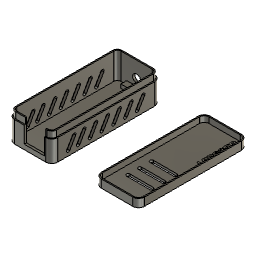
TubesZB_2022_PoE_Coordinator_Case_Rev_K_Olimex (Autodesk Fusion 360 design; units mm, degrees)
Autodesk Fusion 360 part; units mm, degrees
note: some values were not read from the file. Set by a fixed rule: which face or edge a step refers to.
sketch "Sketch1" plane through (0, 0, 0) normal (0, 0, 1) x (1, 0, 0)
  line L0 (0, 0) -> (36.6, 0)
  line L1 (36.6, 0) -> (36.6, 92.2)
  line L2 (36.6, 92.2) -> (0, 92.2)
  line L3 (0, 92.2) -> (0, 0)
  line L4 (105.8273, 96.6) -> (69.2273, 96.6)
  line L5 (69.2273, 4.4) -> (105.8273, 4.4)
  line L6 (105.8273, 4.4) -> (105.8273, 96.6)
  line L7 (69.2273, 96.6) -> (69.2273, 4.4)
  dimension "d1" = 36.6
  dimension "d2" = 92.2
  dimension "d3" = 36.6
  dimension "d4" = 92.2
  constraint horizontal L0
  constraint vertical L1
  constraint horizontal L2
  constraint vertical L3
  constraint coincident L0.start L3.end
  constraint horizontal L5
  constraint vertical L6
  constraint horizontal L4
  constraint vertical L7
  measures "d1" distance of L0.start L0.end
  measures "d2" distance of L0.start L2.end
  measures "d3" distance of L5.start L5.end
  measures "d4" distance of L4.end L5.start
extrude "Extrude1" add sketch "Sketch1" along normal blind 18 contours L0 L1 L2 L3 makes body 1
sketch "Sketch2" plane through (0, 0, 0) normal (0, 0, 1) x (1, 0, 0)
extrude "Extrude2" add sketch "Sketch1" along normal blind 6.8 separate body contours L4 L5 L6 L7 makes body 2
fillet "Fillet1" radius 5 4 edges at (0, 0, 9) (36.6, 0, 9) (36.6, 92.2, 9) (0, 92.2, 9) on bodies 1
fillet "Fillet2" radius 5 4 edges at (105.8273, 4.4, 3.4) (69.2273, 4.4, 3.4) (105.8273, 96.6, 3.4) (69.2273, 96.6, 3.4) on bodies 2
shell "Shell1" thickness 1 removed faces 1 at (93.6273, 36.8, 6.8) on bodies 2
shell "Shell2" thickness 1 removed faces 1 at (12.2, 59.8, 18) on bodies 1
extrude "Extrude3" cut 1 faces at (81.7606, 36.8, 1) along direction (0, 0, -1) blind 0.1 on bodies 2 bodies 2
extrude "Extrude4" add 1 faces at (12.5333, 59.8, 1) along direction (0, 0, 1) blind 22.2 on bodies 1 bodies 1
shell "Shell3" thickness 1 removed faces 1 at (12.5333, 59.8, 23.2) on bodies 1
extrude "Extrude5" cut 1 faces at (12.5333, 59.8, 1) along direction (0, 0, -1) blind 0.1 on bodies 1 bodies 1
sketch "Sketch3" plane through (36.6, 0, 0) normal (1, 0, 0) x (0, 1, 0)
  line L0 (87.2, 0) -> (87.2, 18)
  line L1 (87.2, 18) -> (5, 18)
  line L2 (5, 18) -> (5, 0)
  line L3 (5, 0) -> (87.2, 0)
  line L4 (15.2859, 3.55) -> (20.2859, 12.2103)
  arc A0 (20.2859, 12.2103) -> (17.6878, 13.7103) centre (18.9869, 12.9603) ccw
  line L5 (17.6878, 13.7103) -> (12.6878, 5.05)
  arc A1 (12.6878, 5.05) -> (15.2859, 3.55) centre (13.9869, 4.3) ccw
  line L6 (13.9869, 4.3) -> (18.9869, 12.9603) construction
  arc A2 (21.1822, 5.05) -> (23.7803, 3.55) centre (22.4812, 4.3) ccw
  arc A3 (28.7803, 12.2103) -> (26.1822, 13.7103) centre (27.4812, 12.9603) ccw
  line L7 (22.4812, 4.3) -> (27.4812, 12.9603) construction
  line L8 (23.7803, 3.55) -> (28.7803, 12.2103)
  line L9 (26.1822, 13.7103) -> (21.1822, 5.05)
  arc A4 (38.7803, 12.2103) -> (36.1822, 13.7103) centre (37.4812, 12.9603) ccw
  line L10 (33.7803, 3.55) -> (38.7803, 12.2103)
  line L11 (32.4812, 4.3) -> (37.4812, 12.9603) construction
  arc A5 (31.1822, 5.05) -> (33.7803, 3.55) centre (32.4812, 4.3) ccw
  line L12 (36.1822, 13.7103) -> (31.1822, 5.05)
  line L13 (43.7803, 3.55) -> (48.7803, 12.2103)
  line L14 (46.1822, 13.7103) -> (41.1822, 5.05)
  line L15 (42.4812, 4.3) -> (47.4812, 12.9603) construction
  arc A6 (41.1822, 5.05) -> (43.7803, 3.55) centre (42.4812, 4.3) ccw
  arc A7 (48.7803, 12.2103) -> (46.1822, 13.7103) centre (47.4812, 12.9603) ccw
  line L16 (53.7803, 3.55) -> (58.7803, 12.2103)
  arc A8 (51.1822, 5.05) -> (53.7803, 3.55) centre (52.4812, 4.3) ccw
  line L17 (52.4812, 4.3) -> (57.4812, 12.9603) construction
  arc A9 (58.7803, 12.2103) -> (56.1822, 13.7103) centre (57.4812, 12.9603) ccw
  line L18 (56.1822, 13.7103) -> (51.1822, 5.05)
  line L19 (63.7803, 3.55) -> (68.7803, 12.2103)
  line L20 (62.4812, 4.3) -> (67.4812, 12.9603) construction
  line L21 (66.1822, 13.7103) -> (61.1822, 5.05)
  arc A10 (68.7803, 12.2103) -> (66.1822, 13.7103) centre (67.4812, 12.9603) ccw
  arc A11 (61.1822, 5.05) -> (63.7803, 3.55) centre (62.4812, 4.3) ccw
  arc A12 (71.1822, 5.05) -> (73.7803, 3.55) centre (72.4812, 4.3) ccw
  arc A13 (78.7803, 12.2103) -> (76.1822, 13.7103) centre (77.4812, 12.9603) ccw
  line L22 (76.1822, 13.7103) -> (71.1822, 5.05)
  line L23 (73.7803, 3.55) -> (78.7803, 12.2103)
  line L24 (72.4812, 4.3) -> (77.4812, 12.9603) construction
  point P0 (38.7803, 12.2103)
  dimension "d22" = 10
  dimension "d23" = 3
  dimension "d24" = 10
  dimension "d25" = 3
  dimension "d26" = 10
  dimension "d27" = 3
  dimension "d28" = 10
  dimension "d29" = 3
  dimension "d30" = 10
  dimension "d31" = 3
  dimension "d32" = 10
  dimension "d33" = 3
  dimension "d34" = 10
  dimension "d35" = 3
  constraint tangent L4 A0
  constraint tangent A0 L5
  constraint parallel L4 L5
  constraint tangent L5 A1
  constraint tangent L4 A1
  constraint tangent A3 L8
  constraint tangent A3 L9
  constraint parallel L8 L9
  constraint tangent A2 L9
  constraint tangent A2 L8
  constraint tangent A4 L10
  constraint tangent A4 L12
  constraint parallel L10 L12
  constraint tangent A5 L12
  constraint tangent L10 A5
  constraint tangent L13 A7
  constraint tangent L14 A7
  constraint parallel L13 L14
  constraint tangent L14 A6
  constraint tangent L13 A6
  constraint tangent L16 A9
  constraint tangent A9 L18
  constraint parallel L16 L18
  constraint tangent A8 L18
  constraint tangent L16 A8
  constraint tangent L19 A10
  constraint tangent L21 A10
  constraint parallel L19 L21
  constraint tangent L21 A11
  constraint tangent L19 A11
  constraint tangent A13 L23
  constraint tangent A13 L22
  constraint parallel L22 L23
  constraint tangent A12 L22
  constraint tangent A12 L23
  measures "d22" distance of A1.centre A0.centre
  measures "d23" diameter of A0
  measures "d24" distance of A2.centre A3.centre
  measures "d25" diameter of A3
  measures "d26" distance of A4.centre L11.start
  measures "d27" diameter of A4
  measures "d28" distance of L15.start L15.end
  measures "d29" diameter of A7
  measures "d30" distance of L17.end A8.centre
  measures "d31" diameter of A9
  measures "d32" distance of L20.start L20.end
  measures "d33" diameter of A10
  measures "d34" distance of A12.centre A13.centre
  measures "d35" diameter of A13
extrude "Extrude13" cut sketch "Sketch3" against normal blind 59.488 contours L4 A0 L5 A1 | A2 A3 L8 L9 | A4 L10 A5 L12 | L13 L14 A6 A7 | L16 A8 A9 L18 | L19 L21 A10 A11 | A12 A13 L22 L23 bodies 1
sketch "Sketch4" plane through (0, 0, 0.9) normal (0, 0, 1) x (-1, 0, 0)
  arc A0 (-74.2273, -95.6) -> (-70.2273, -91.6) centre (-74.2273, -91.6) ccw
  line L0 (-70.2273, -91.6) -> (-70.2273, -9.4)
  arc A1 (-70.2273, -9.4) -> (-74.2273, -5.4) centre (-74.2273, -9.4) ccw
  line L1 (-74.2273, -5.4) -> (-100.8273, -5.4)
  arc A2 (-100.8273, -5.4) -> (-104.8273, -9.4) centre (-100.8273, -9.4) ccw
  line L2 (-104.8273, -9.4) -> (-104.8273, -91.6)
  arc A3 (-104.8273, -91.6) -> (-100.8273, -95.6) centre (-100.8273, -91.6) ccw
  line L3 (-100.8273, -95.6) -> (-74.2273, -95.6)
  line L4 (-77.8, -22.0707) -> (-97.8, -22.0707)
  arc A4 (-97.8, -22.0707) -> (-97.8, -25.0707) centre (-97.8, -23.5707) ccw
  line L5 (-97.8, -25.0707) -> (-77.8, -25.0707)
  arc A5 (-77.8, -25.0707) -> (-77.8, -22.0707) centre (-77.8, -23.5707) ccw
  line L6 (-77.8, -23.5707) -> (-97.8, -23.5707) construction
  line L7 (-77.8, -32.0707) -> (-97.8, -32.0707)
  arc A6 (-97.8, -32.0707) -> (-97.8, -35.0707) centre (-97.8, -33.5707) ccw
  line L8 (-97.8, -35.0707) -> (-77.8, -35.0707)
  arc A7 (-77.8, -35.0707) -> (-77.8, -32.0707) centre (-77.8, -33.5707) ccw
  line L9 (-77.8, -33.5707) -> (-97.8, -33.5707) construction
  line L10 (-77.8, -43.5707) -> (-97.8, -43.5707) construction
  line L11 (-97.8, -45.0707) -> (-77.8, -45.0707)
  arc A8 (-77.8, -45.0707) -> (-77.8, -42.0707) centre (-77.8, -43.5707) ccw
  line L12 (-77.8, -42.0707) -> (-97.8, -42.0707)
  arc A9 (-97.8, -42.0707) -> (-97.8, -45.0707) centre (-97.8, -43.5707) ccw
  constraint tangent L4 A4
  constraint tangent A4 L5
  constraint parallel L4 L5
  constraint tangent L5 A5
  constraint tangent L4 A5
  constraint horizontal L6
  constraint tangent L7 A6
  constraint tangent A6 L8
  constraint parallel L7 L8
  constraint tangent L8 A7
  constraint tangent L7 A7
  constraint horizontal L9
  constraint tangent L12 A9
  constraint tangent L11 A9
  constraint parallel L11 L12
  constraint tangent L11 A8
  constraint tangent A8 L12
  constraint horizontal L10
extrude "Extrude7" cut sketch "Sketch4" against normal blind 5 contours L4 A4 L5 A5 | L7 A6 L8 A7 | L11 A8 L12 A9 bodies 2
sketch "Sketch5" plane through (0, 0, 0) normal (0, 0, 1) x (1, 0, 0)
  line L0 (98.3981, 60.428) -> (98.2294, 82.6189) construction
  line L1 (98.2294, 82.6189) -> (102.261, 82.6495) construction
  line L2 (102.261, 82.6495) -> (102.4296, 60.4586) construction
  line L3 (102.4296, 60.4586) -> (98.3981, 60.428) construction
  dimension "d41" = 5
  text T0 "TubesZB" font "Arial Black" height 5 align left top in box 22.1915 x 4.0317 at (98.3981, 60.428) x (-0.007601, 0.999971) y (0.999971, 0.007601) spacing 1
extrude "Extrude8" add 1 faces at (84.2849, 76.0902, 0.9) along direction (0, 0, 1) blind 1 on bodies 2 bodies 2
extrude "Extrude9" cut sketch "Sketch5" along normal blind 1.6 text T0 bodies 2
sketch "Sketch6" plane through (0, 0, 0) normal (0, 1, 0) x (1, 0, 0)
  line L0 (13.2509, -4) -> (30.4509, -4)
  line L1 (30.4509, -4) -> (30.4509, -25.23)
  line L2 (30.4509, -25.23) -> (13.2509, -25.23)
  line L3 (13.2509, -25.23) -> (13.2509, -4)
  dimension "d46" = 17.2
  dimension "d47" = 21.23
  constraint horizontal L0
  constraint vertical L1
  constraint horizontal L2
  constraint vertical L3
  measures "d46" distance of L0.start L0.end
  measures "d47" distance of L0.start L2.end
extrude "Extrude10" add 1 faces at (1.3333, 59.8, 23.2) along direction (0, 0, -1) blind 23 on bodies 1 bodies 1
extrude "Extrude11" cut sketch "Sketch3" against normal blind 49.34 contours L4 A0 L5 A1 | A2 A3 L8 L9 | A4 L10 A5 L12 | L13 L14 A6 A7 | L16 A8 A9 L18 | L19 L21 A10 A11 | A12 A13 L22 L23 bodies 1
extrude "Extrude12" cut sketch "Sketch6" along normal blind 6.725 bodies 1
sketch "Sketch7" plane through (0, 0, 0.9) normal (0, 0, 1) x (-1, 0, 0)
  arc A0 (-31.6, -2) -> (-34.6, -5) centre (-31.6, -5) ccw
  line L0 (-34.6, -5) -> (-34.6, -87.2)
  arc A1 (-34.6, -87.2) -> (-31.6, -90.2) centre (-31.6, -87.2) ccw
  line L1 (-31.6, -90.2) -> (-5, -90.2)
  arc A2 (-5, -90.2) -> (-2, -87.2) centre (-5, -87.2) ccw
  line L2 (-2, -87.2) -> (-2, -5)
  arc A3 (-2, -5) -> (-5, -2) centre (-5, -5) ccw
  line L3 (-5, -2) -> (-31.6, -2)
  line L4 (-9.9766, -90.2) -> (-27.9766, -90.2)
  line L5 (-27.9766, -90.2) -> (-27.9766, -85.2)
  line L6 (-27.9766, -85.2) -> (-9.9766, -85.2)
  line L7 (-9.9766, -85.2) -> (-9.9766, -90.2)
  dimension "d56" = 18
  dimension "d57" = 5
  constraint horizontal L4
  constraint vertical L5
  constraint horizontal L6
  constraint vertical L7
  constraint coincident L1 L4.start
  measures "d56" distance of L4.start L4.end
  measures "d57" distance of L4.start L6.end
extrude "Extrude14" add sketch "Sketch7" along normal blind 3.1 contours L1 L4 L5 L6 L7 bodies 1
sketch "Sketch8" plane through (0, 92.2, 0) normal (0, 1, 0) x (-1, 0, 0)
  line L0 (-5, 0) -> (-5, 18)
  line L1 (-5, 18) -> (-31.6, 18)
  line L2 (-31.6, 18) -> (-31.6, 0)
  line L3 (-31.6, 0) -> (-5, 0)
  circle A0 centre (-18.3, 9.6573) radius 3.4
  dimension "d60" = 6.8
  measures "d60" diameter of A0
extrude "Extrude15" cut sketch "Sketch8" against normal blind 3.069 contours A0 bodies 1
